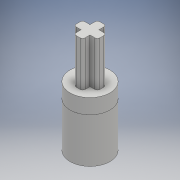
# Autodesk Inventor part: Motor_Axle_Adapter
Saved by Autodesk Inventor 2018.2 (Build 222227000, 227)
## iProperties
Created: 2018-08-11
Part Number: Motor_Axle_Adapter
Material: Generic
Document SubType Name: Modeling
Designer: mateu
Density: 1 g/cm^3
Appearance: Default
Author: mateu
Autodesk Inventor part; units mm, degrees
ref_plane "YZ Plane" through (0, 0, 0) normal (1, 0, 0) x (0, 1, 0)
ref_plane "XZ Plane" through (0, 0, 0) normal (0, 1, 0) x (-1, 0, 0)
ref_plane "XY Plane" through (0, 0, 0) normal (0, 0, 1) x (1, 0, 0)
sketch "Sketch1" plane through (0, 0, 0) normal (0, 0, 1) x (1, 0, 0)
  circle A0 centre (0, 0) radius 2.125
  circle A1 centre (0, 0) radius 4
  dimension "d0" = 4.25
  dimension "d1" = 8
  constraints: 2 centre point, 2 coincident
  measures "d0" diameter of A0
  measures "d1" diameter of A1
extrude "Extrusion1" add sketch "Sketch1" along normal blind 9
sketch "Sketch2" plane through (0, 0, 9) normal (0, 0, 1) x (1, 0, 0)
  circle A0 centre (0, 0) radius 4.0023
  constraints: 1 centre point, 1 coincident
extrude "Extrusion2" add sketch "Sketch2" along normal blind 3
sketch "Sketch3" plane through (0, 0, 12) normal (0, 0, 1) x (1, 0, 0)
  line L0 (2.4, 0.9) -> (2.4, -0.9)
  line L1 (-2.4, -0.9) -> (-2.4, 0.9)
  line L2 (-0.9, 2.4) -> (0.9, 2.4)
  line L3 (0.9, -2.4) -> (-0.9, -2.4)
  line L4 (-0.9, 2.4) -> (-0.9, 0.9)
  line L5 (-0.9, -2.4) -> (-0.9, -0.9)
  line L6 (0.9, 2.4) -> (0.9, 0.9)
  line L7 (0.9, -2.4) -> (0.9, -0.9)
  line L8 (2.4, -0.9) -> (0.9, -0.9)
  line L9 (-0.9, -0.9) -> (-2.4, -0.9)
  line L10 (-2.4, 0.9) -> (-0.9, 0.9)
  line L11 (0.9, 0.9) -> (2.4, 0.9)
  point P0 (0, 0)
  dimension "d6" = 4.8
  dimension "d7" = 1.8
  dimension "d8" = 2.4
  dimension "d10" = 1.8
  dimension "d11" = 4.8
  dimension "d12" = 2.4
  constraints: 24 end point, 5 equal length, 2 horizontal, 2 point on line
  measures "d6" distance of L0.end L1.start
  measures "d7" distance of L0.start L0.end
  measures "d8" distance from line of point (0, 0) L1
  measures "d10" distance of L3.start L3.end
  measures "d11" distance of L2.end L3.start
  measures "d12" distance from line of L2 point (0, 0)
extrude "Extrusion3" add sketch "Sketch3" along normal blind 9
sketch "Sketch4" plane through (0, 0, 0) normal (0, 0, -1) x (-1, 0, 0)
  line L0 (0, 1.475) -> (1.5297, 1.475)
  line L1 (-1.5297, 1.475) -> (0, 1.475)
  arc A0 (1.5297, 1.475) -> (-1.5297, 1.475) centre (0, 0) ccw
  point P0 (0, 0)
  constraints: 4 end point, 2 point on circle, 1 centre point, 1 collinear, 1 horizontal, 1 point on line
fillet "Fillet1" radius 0.5 2 edges at (-0.9, 2.4, 16.5) (-2.4, 0.9, 16.5)
fillet "Fillet2" radius 0.5 1 edges at (-2.4, -0.9, 16.5)
fillet "Fillet3" radius 0.5 1 edges at (-0.9, -2.4, 16.5)
fillet "Fillet4" radius 0.5 4 edges at (0.9, 2.4, 16.5) (2.4, 0.9, 16.5) (2.4, -0.9, 16.5) (0.9, -2.4, 16.5)
body "Solid1"
